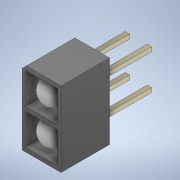
# Autodesk Inventor part: LBR-127
Saved by Autodesk Inventor 2022 (Build 260153000, 153)
## iProperties
Created: 2024-06-24
Part Number: LBR-127
Material: 一般
Document SubType Name: Modeling
Designer: yamashita1
Density: 1 g/cm^3
Appearance: 既定
Author: yamashita1
Autodesk Inventor part; units mm, degrees
ref_plane "YZ Plane" through (0, 0, 0) normal (1, 0, 0) x (0, 1, 0)
ref_plane "XZ Plane" through (0, 0, 0) normal (0, 1, 0) x (-1, 0, 0)
ref_plane "XY Plane" through (0, 0, 0) normal (0, 0, 1) x (1, 0, 0)
sketch "スケッチ1" plane through (0, 0, 0) normal (0, 0, 1) x (1, 0, 0)
  line L0 (-2.25, 4.35) -> (2.25, 4.35)
  line L1 (2.25, 4.35) -> (2.25, -4.35)
  line L2 (2.25, -4.35) -> (-2.25, -4.35)
  line L3 (-2.25, -4.35) -> (-2.25, 4.35)
  line L4 (-3.4568, 2.05) -> (3.4568, 2.05) construction
  line L5 (3.4568, -2.05) -> (-3.4568, -2.05) construction
  line L6 (-4.4106, 0) -> (4.4106, 0) construction
  line L7 (-1.85, 3.85) -> (1.85, 3.85)
  line L8 (1.85, 3.85) -> (1.85, 0.25)
  line L9 (1.85, 0.25) -> (-1.85, 0.25)
  line L10 (-1.85, 0.25) -> (-1.85, 3.85)
  line L11 (-1.85, -0.25) -> (1.85, -0.25)
  line L12 (1.85, -0.25) -> (1.85, -3.85)
  line L13 (1.85, -3.85) -> (-1.85, -3.85)
  line L14 (-1.85, -3.85) -> (-1.85, -0.25)
  line L15 (-1.75, 4.35) -> (-2.25, 3.85)
  circle A0 centre (0, 2.05) radius 1.45
  circle A1 centre (0, -2.05) radius 1.45
  line L16 (1.27, 5.4107) -> (1.27, -6.214) construction
  line L17 (-1.27, -6.214) -> (-1.27, 5.4107) construction
  line L18 (0, 6.0924) -> (0, -6.0924) construction
  line L19 (1.52, 2.3) -> (1.02, 2.3)
  line L20 (1.02, 2.3) -> (1.02, 1.8)
  line L21 (1.02, 1.8) -> (1.52, 1.8)
  line L22 (1.52, 1.8) -> (1.52, 2.3)
  line L23 (-1.02, 2.3) -> (-1.52, 2.3)
  line L24 (-1.52, 2.3) -> (-1.52, 1.8)
  line L25 (-1.52, 1.8) -> (-1.02, 1.8)
  line L26 (-1.02, 1.8) -> (-1.02, 2.3)
  line L27 (1.52, -1.8) -> (1.02, -1.8)
  line L28 (1.02, -1.8) -> (1.02, -2.3)
  line L29 (1.02, -2.3) -> (1.52, -2.3)
  line L30 (1.52, -2.3) -> (1.52, -1.8)
  line L31 (-1.02, -1.8) -> (-1.52, -1.8)
  line L32 (-1.52, -1.8) -> (-1.52, -2.3)
  line L33 (-1.52, -2.3) -> (-1.02, -2.3)
  line L34 (-1.02, -2.3) -> (-1.02, -1.8)
  point P0 (0, 0)
  point P1 (0, 4.35)
  point P2 (-2.25, 0)
  point P3 (0, 0)
  point P4 (-1.85, 2.05)
  point P5 (0, 3.85)
  point P6 (1.85, -2.05)
  point P7 (0, -3.85)
  point P8 (1.27, 2.3)
  point P9 (1.52, 2.05)
  point P10 (-1.27, 2.3)
  point P11 (-1.52, 2.05)
  point P12 (1.27, -1.8)
  point P13 (1.52, -2.05)
  point P14 (-1.27, -1.8)
  dimension "d0" = 4.5
  dimension "d1" = 8.7
  dimension "d2" = 4.1
  dimension "d3" = 3.7
  dimension "d4" = 3.6
  dimension "d5" = 0.5
  dimension "d6" = 0.5
  dimension "d9" = 2.9
  dimension "d13" = 2.54
  dimension "d14" = 0.5
  constraints: 70 end point, 17 midpoint, 14 parallel, 13 point on line, 8 equal length, 8 horizontal, 7 perpendicular, 5 vertical alignment, 2 centre point, 2 vertical, 1 coincident, 1 equal radius, 1 horizontal alignment, 2 other
  measures "d0" distance of L1.end L2.end
  measures "d1" distance of L0.end L1.end
  measures "d2" distance between parallel lines of L5 L4
  measures "d3" distance of L8.end L9.end
  measures "d4" distance of L7.end L8.end
  measures "d5" distance of L0.start L15.start
  measures "d6" distance of L0.start L15.end
  measures "d9" diameter of A0
  measures "d13" distance between parallel lines of L17 L16
  measures "d14" distance of L19.start L19.end
extrude "押し出し1" add sketch "スケッチ1" along normal blind 5.6 contours L0 L1 L2 L3 L15
extrude "押し出し2" add sketch "スケッチ1" along normal blind 5.6 contours A0 L21 L20 L19 | L19 L20 L21 A0 L25 L26 L23 | L23 L26 L25 A0 | A1 L29 L28 L27 | L27 L28 L29 A1 L33 L34 L31 | L31 L34 L33 A1
fillet "フィレット1" radius 1.45 2 edges at (-1.45, 2.05, 5.6) (-1.45, -2.05, 5.6)
extrude "押し出し3" add sketch "スケッチ1" against normal blind 5.6 contours A0 L21 L20 L19 | A0 L19 L22 L21 | L23 L26 L25 A0 | A0 L25 L24 L23 | A1 L29 L28 L27 | A1 L27 L30 L29 | L31 L34 L33 A1 | A1 L33 L32 L31
extrude "押し出し4" add sketch "スケッチ1" along normal blind 0.5 contours L7 L8 L9 L10 | L11 L12 L13 L14 | A0 L21 L20 L19 | A0 L19 L22 L21 | L19 L20 L21 A0 L25 L26 L23 | L23 L26 L25 A0 | A0 L25 L24 L23 | A1 L29 L28 L27 | A1 L27 L30 L29 | L27 L28 L29 A1 L33 L34 L31 | L31 L34 L33 A1 | A1 L33 L32 L31
equation "\"d6\" = d5"
